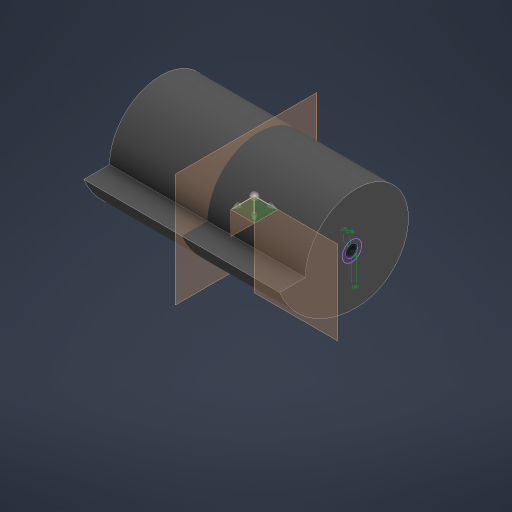
# Autodesk Inventor part: Drum
Saved by Autodesk Inventor 2024.1 (Build 281209000, 209)
## iProperties
Created: 2023-10-18
Part Number: Drum
Material: Generic
Document SubType Name: Modeling
Designer: CJ110
Density: 1 g/cm^3
Appearance: Default
Mass: 194.247 g
Surface Area: 207.239 cm^2
Volume: 194.247 cm^3
Author: CJ110
Autodesk Inventor part; units mm, degrees
ref_plane "YZ Plane" through (0, 0, 0) normal (1, 0, 0) x (0, 1, 0)
ref_plane "XZ Plane" through (0, 0, 0) normal (0, 1, 0) x (-1, 0, 0)
ref_plane "XY Plane" through (0, 0, 0) normal (0, 0, 1) x (1, 0, 0)
sketch "Sketch1" plane through (0, 0, 0) normal (0, 1, 0) x (-1, 0, 0)
  circle A0 centre (0, 0) radius 25.4
  line L0 (0, 25.4) -> (0, 38.1)
  line L1 (0, 0) -> (0, 25.4) construction
  arc A1 (0, 38.1) -> (-25.4, 0) centre (15.875, 0) ccw
  line L2 (0, 0) -> (-25.4, 0) construction
  dimension "d0" = 50.8
  dimension "d1" = 12.7
  constraints: 6 end point, 5 point on circle, 2 centre point, 2 vertical, 1 coincident, 1 collinear, 1 horizontal, 1 tangent
  measures "d0" diameter of A0
  measures "d1" distance of L0.start L0.end
extrude "Extrusion1" add sketch "Sketch1" along normal blind 96.52
ref_plane "Work Plane1" through (0, 48.26, 0) normal (0, 1, 0) x (1, 0, 0)
sketch "Sketch2" plane through (0, 96.52, 0) normal (0, 1, 0) x (1, 0, 0)
  circle A0 centre (0, -2.54) radius 2.921
  circle A1 centre (0, -2.54) radius 4.7625
  circle A2 centre (0, -2.54) radius 2.286
  point P0 (0, 0)
  dimension "d4" = 2.54
  dimension "d5" = 5.842
  dimension "d6" = 9.525
  dimension "d11" = 4.572
  constraints: 3 centre point, 2 coincident
  measures "d4" distance of point (0, 0) A0.centre
  measures "d5" diameter of A0
  measures "d6" diameter of A1
  measures "d11" diameter of A2
extrude "Extrusion2" add sketch "Sketch2" against normal blind 12.7 from surface at -96.52 contours A0 | A1 | A2
extrude "Extrusion3" cut sketch "Sketch2" against normal blind 13.97 contours A0 | A2
body "Solid1"
